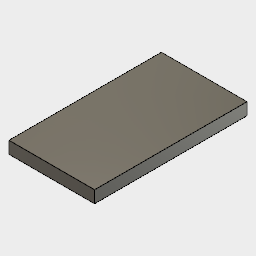
LiPo1200mAh v1 (Autodesk Fusion 360 design; units mm, degrees)
Autodesk Fusion 360 part; units mm, degrees
box "BoxPrimitive1" add length 60.5 width 34 height 4.85 placed x (0, 0, -1) y (-1, 0, 0) z (0, 1, 0) at (-47.8163, 0, 0)
move_body "MoveBody1" bodies 1 to x (1, 0, 0) y (0, 1, 0) z (0, 0, 1) at (45, 0, 0)
